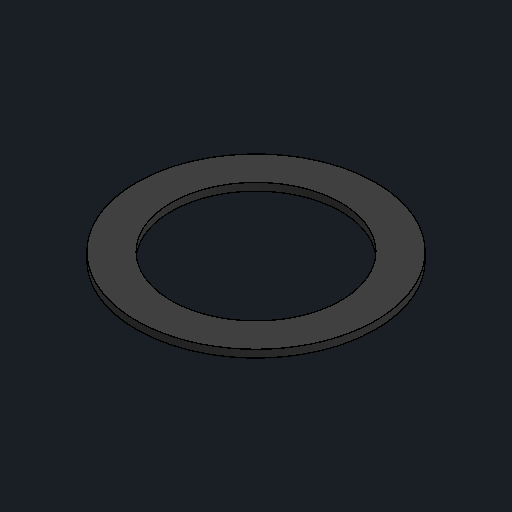
# Autodesk Inventor part: Cylone Adapter Sealing Gasket
Saved by Autodesk Inventor 2026.2 (Build 302298000, 298)
## iProperties
Created: 2026-06-17
Part Number: Cylone Adapter Sealing Gasket
Material: Rubber
Document SubType Name: Modeling
Designer: JoshuaEah
Density: 0.93 g/cm^3
Appearance: Rubber - Black
Author: JoshuaEah
Autodesk Inventor part; units mm, degrees
ref_plane "YZ Plane" through (0, 0, 0) normal (1, 0, 0) x (0, 1, 0)
ref_plane "XZ Plane" through (0, 0, 0) normal (0, 1, 0) x (-1, 0, 0)
ref_plane "XY Plane" through (0, 0, 0) normal (0, 0, 1) x (1, 0, 0)
sketch "Sketch1" plane through (0, 0, 0) normal (0, 1, 0) x (-1, 0, 0)
  circle A0 centre (0, 0) radius 11.2
  circle A1 centre (0, 0) radius 15.8
  dimension "d0" = 22.4
  dimension "d1" = 31.6
  constraints: 2 centre point, 2 coincident
  measures "d0" diameter of A0
  measures "d1" diameter of A1
extrude "Extrusion1" add sketch "Sketch1" along normal blind 1
body "Solid1"
